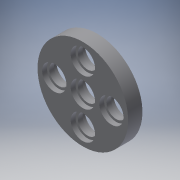
# Autodesk Inventor part: XL320_IdlerToOllo
Saved by Autodesk Inventor 2017 (Build 210142000, 142)
## iProperties
Created: 2014-03-07
Part Number: XL320_IdlerToOllo
Material: Générique
Document SubType Name: Modeling
Designer: Grégoire
Density: 1 g/cm^3
Appearance: Par défaut
Author: Grégoire
Autodesk Inventor part; units mm, degrees
ref_plane "YZ Plane" through (0, 0, 0) normal (1, 0, 0) x (0, 1, 0)
ref_plane "XZ Plane" through (0, 0, 0) normal (0, 1, 0) x (-1, 0, 0)
sketch "Esquisse1" plane through (0, 0, 0) normal (0, 1, 0) x (-1, 0, 0)
  circle A0 centre (0, 0) radius 9.5
  circle A1 centre (0, 0) radius 2.05
  line L0 (0, 9.5) -> (0, -9.5) construction
  line L1 (-9.5, 0) -> (9.5, 0) construction
  circle A2 centre (0, -6) radius 2.05
  circle A3 centre (0, 6) radius 2.05
  circle A4 centre (0, 0) radius 2.05
  circle A5 centre (6, 0) radius 2.05
  circle A6 centre (-6, 0) radius 2.05
  circle A7 centre (0, 0) radius 2.05
  dimension "d0" = 19
  dimension "d1" = 4.1
  dimension "d4" = 6
  dimension "d7" = 6
  dimension "d12" = 6
  dimension "d15" = 6
  constraints: 8 centre point, 4 end point, 4 point on circle, 2 coincident, 2 horizontal, 2 vertical, 1 perpendicular, 12 other
  measures "d0" diameter of A0
  measures "d1" diameter of A1
  measures "d4" distance of A1.centre A2.centre
  measures "d7" distance of A1.centre A3.centre
  measures "d12" distance of A1.centre A5.centre
  measures "d15" distance of A1.centre A6.centre
extrude "Extrusion1" add sketch "Esquisse1" along normal blind 3
sketch "Sketch2" plane through (0, 0, 0) normal (0, -1, 0) x (1, 0, 0)
  circle A0 centre (-6, 0) radius 2.05 projected
  circle A1 centre (-6, 0) radius 2.55
  circle A2 centre (0, 6) radius 2.05 projected
  circle A3 centre (0, 6) radius 2.55
  circle A4 centre (0, 0) radius 2.55
  circle A5 centre (6, 0) radius 2.05 projected
  circle A6 centre (6, 0) radius 2.55
  circle A7 centre (0, -6) radius 2.05 projected
  circle A8 centre (0, -6) radius 2.55
  dimension "d20" = 5.1
  dimension "d21" = 5.1
  dimension "d22" = 5.1
  dimension "d23" = 5.1
  dimension "d24" = 5.1
  constraints: 5 centre point, 5 coincident
  measures "d20" diameter of A1
  measures "d21" diameter of A3
  measures "d22" diameter of A4
  measures "d23" diameter of A6
  measures "d24" diameter of A8
extrude "Extrusion2" cut sketch "Sketch2" against normal blind 1
ref_plane "Work Plane1" through (0, 1.5, 0) normal (0, -1, 0) x (1, 0, 0)
mirror "Mirror1" about plane through (0, 1.5, 0) normal (0, -1, 0) of "Extrusion2"
